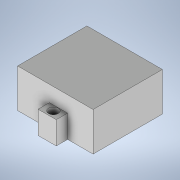
# Autodesk Inventor part: shell
Saved by Autodesk Inventor 2020.2 (Build 242310000, 310)
## iProperties
Created: 2020-02-05
Part Number: shell
Material: Generic
Document SubType Name: Modeling
Designer: ColinP
Density: 1 g/cm^3
Appearance: Default
Author: ColinP
Autodesk Inventor part; units mm, degrees
ref_plane "YZ Plane" through (0, 0, 0) normal (1, 0, 0) x (0, 1, 0)
ref_plane "XZ Plane" through (0, 0, 0) normal (0, 1, 0) x (-1, 0, 0)
ref_plane "XY Plane" through (0, 0, 0) normal (0, 0, 1) x (1, 0, 0)
sketch "Sketch10" plane through (0, 0, 0) normal (0, 1, 0) x (-1, 0, 0)
  line L0 (16.6, 18.8056) -> (-16.6, 18.8056)
  line L1 (-16.6, 18.8056) -> (-16.6, -11.6944)
  line L2 (-16.6, -11.6944) -> (16.5, -11.6944)
  line L3 (16.6, 18.8056) -> (16.6, -11.6944)
  line L4 (16.6, 18.8056) -> (47.1, 18.8056) construction
  line L5 (16.6, -11.6944) -> (16.5, -11.6944)
  point P0 (0, 0)
  dimension "d53" = 33.2
  dimension "d54" = 30.5
  dimension "d55" = 90
  constraints: 12 end point, 3 perpendicular, 2 horizontal, 1 collinear, 1 point on line
  measures "d53" distance of L0.start L0.end
  measures "d54" distance of L0.end L1.end
  measures "d55" angle of L3 L4
extrude "Extrusion8" add sketch "Sketch10" against normal blind 1
sketch "Sketch11" plane through (0, -1, 0) normal (0, -1, 0) x (1, 0, 0)
  line L0 (16.6, 18.8056) -> (-16.6, 18.8056) projected
  line L1 (-16.6, 18.8056) -> (-15.6, 18.8056)
  line L2 (-15.6, 18.8056) -> (-15.6, 17.8056)
  line L3 (-15.6, 17.8056) -> (15.6, 17.8056)
  line L4 (15.6, 17.8056) -> (15.6, -10.6944)
  line L5 (16.6, -11.6944) -> (16.6, 18.8056) projected
  line L6 (15.6, -10.6944) -> (-15.6, -10.6944)
  line L7 (-15.6, -10.6944) -> (-15.6, 17.8056)
  line L8 (-16.6, -11.6944) -> (16.6, -11.6944) projected
  line L9 (16.6, -11.6944) -> (16.6, 18.8056) projected
  line L10 (16.6, 18.8056) -> (-16.6, 18.8056) projected
  line L11 (-16.6, 18.8056) -> (-16.6, -11.6944) projected
  point P0 (0, 0)
  dimension "d58" = 1
  dimension "d59" = 1
  dimension "d60" = 31.2
  dimension "d61" = 28.5
  dimension "d62" = 90
  constraints: 12 end point, 4 perpendicular, 2 point on line, 1 parallel
  measures "d58" distance of L0.end L1.end
  measures "d59" distance of L1.end L2.end
  measures "d60" distance of L2.end L3.end
  measures "d61" distance of L3.end L4.end
  measures "d62" angle of L3 L4
extrude "Extrusion9" add sketch "Sketch11" along normal blind 16
sketch "Sketch12" plane through (0, -17, 0) normal (0, -1, 0) x (1, 0, 0)
  point P0 (0, 0)
sketch "Sketch13" plane through (0, -17, 0) normal (0, -1, 0) x (1, 0, 0)
  line L0 (-16.6, -11.6944) -> (-16.6, 18.8056) projected
  line L1 (-16.6, 3.5556) -> (1.4, 3.5556)
  line L2 (1.4, 3.5556) -> (1.4, 21.0556)
  line L3 (1.4, 21.0556) -> (1.4, -13.9444)
  circle A0 centre (1.4, 21.0556) radius 2.1
  circle A1 centre (1.4, -13.9444) radius 2.1
  line L4 (-16.6, 18.8056) -> (16.6, 18.8056) projected
  line L5 (1.4, 18.8056) -> (5.4, 18.8056)
  line L6 (5.4, 18.8056) -> (5.4, 23.8056)
  line L7 (5.4, 23.8056) -> (-2.6, 23.8056)
  line L8 (-2.6, 23.8056) -> (-2.6, 18.8056)
  line L9 (16.6, -11.6944) -> (-16.6, -11.6944) projected
  line L10 (5.4, -11.6944) -> (5.4, -16.6944)
  line L11 (5.4, -16.6944) -> (-2.6, -16.6944)
  line L12 (-2.6, -16.6944) -> (-2.6, -11.6944)
  point P0 (0, 0)
  dimension "d65" = 18
  dimension "d66" = 17.5
  dimension "d67" = 35
  dimension "d68" = 4.2
  dimension "d69" = 4.2
  dimension "d70" = 4
  dimension "d71" = 5
  dimension "d72" = 90
  dimension "d73" = 8
  dimension "d74" = 5
  constraints: 20 end point, 11 point on line, 5 perpendicular, 2 centre point, 2 coincident, 1 horizontal, 1 midpoint
  measures "d65" distance of L1.start L1.end
  measures "d66" distance of L1.end L2.end
  measures "d67" distance of L2.end L3.end
  measures "d68" diameter of A0
  measures "d69" diameter of A1
  measures "d70" distance of L5.start L5.end
  measures "d71" distance of L5.end L6.end
  measures "d72" angle of L6 L5
  measures "d73" distance of L6.end L7.end
  measures "d74" distance of L10.start L10.end
extrude "Extrusion10" add sketch "Sketch13" against normal blind 10 contours L9 L10 L11 L12 | L8 L7 L6 L4
body "Solid3"
